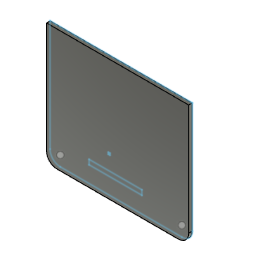
OSSM PCB Case (Autodesk Fusion 360 archive; units mm, degrees)
design "OSSM_PCB"
Autodesk Fusion 360 part; units mm, degrees
sketch "sketch 373" plane through (0, -49.5, 0) normal (0, -1, 0) x (1, 0, 0)
  line L0 (-34.6, -85.0111) -> (-34.6, -31.0111)
  arc A0 (-34.6, -85.0111) -> (-29.6, -90.0111) centre (-29.6, -85.0111) ccw
  line L1 (29.552, -90.0111) -> (-29.6, -90.0111)
  arc A1 (29.552, -90.0111) -> (34.552, -85.0111) centre (29.552, -85.0111) ccw
  line L2 (34.552, -31.0111) -> (34.552, -85.0111)
  line L3 (-34.6, -31.0111) -> (34.552, -31.0111)
extrude "Extrusion1" add sketch "sketch 373" along normal blind 1.7
sketch "sketch 405" plane through (0, -49.5, 15) normal (0, 1, 0) x (-1, 0, 0)
  line L0 (15.6, -97.1111) -> (-10.1, -97.1111)
  line L1 (15.6, -94.8111) -> (15.6, -97.1111)
  line L2 (-10.1, -94.8111) -> (15.6, -94.8111)
  line L3 (-10.1, -97.1111) -> (-10.1, -94.8111)
extrude "Extrusion2" add sketch "sketch 405" along normal blind 8.41
sketch "sketch 426" plane through (0, -41.09, 15) normal (0, 1, 0) x (-1, 0, 0)
  line L0 (14.65, -96.3611) -> (14.65, -95.5611)
  line L1 (14.65, -95.5611) -> (13.85, -95.5611)
  line L2 (13.85, -95.5611) -> (13.85, -96.3611)
  line L3 (13.85, -96.3611) -> (14.65, -96.3611)
extrude "Extrusion3" cut sketch "sketch 426" against normal blind 7
